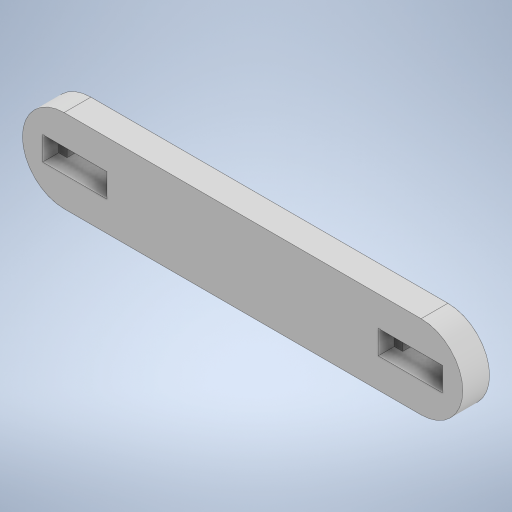
# Autodesk Inventor part: arm 2 right
Saved by Autodesk Inventor 2023 (Build 270158000, 158)
## iProperties
Created: 2024-06-28
Part Number: arm 2 right
Material: Generic
Document SubType Name: Modeling
Designer: Swoby
Density: 1 g/cm^3
Appearance: Default
Author: Swoby
Autodesk Inventor part; units mm, degrees
ref_plane "YZ Plane" through (0, 0, 0) normal (1, 0, 0) x (0, 1, 0)
ref_plane "XZ Plane" through (0, 0, 0) normal (0, 1, 0) x (-1, 0, 0)
ref_plane "XY Plane" through (0, 0, 0) normal (0, 0, 1) x (1, 0, 0)
sketch "Sketch1" plane through (0, 0, 0) normal (0, 0, 1) x (1, 0, 0)
  line L0 (-150, 0) -> (150, 0) construction
  line L1 (-150, -35) -> (150, -35)
  line L2 (150, 35) -> (-150, 35)
  arc A0 (-150, 35) -> (-150, -35) centre (-150, 0) ccw
  arc A1 (150, -35) -> (150, 35) centre (150, 0) ccw
  point P0 (0, 0)
  dimension "d0" = 150
  dimension "d1" = 70
  constraints: 8 end point, 4 point on circle, 4 tangent, 2 centre point, 1 horizontal, 1 midpoint, 1 parallel
  measures "d0" distance of point (0, 0) L0.end
  measures "d1" diameter of A1
extrude "Extrusion1" add sketch "Sketch1" along normal blind 22.5
sketch "Sketch2" plane through (0, 0, 22.5) normal (0, 0, 1) x (1, 0, 0)
  arc A0 (150, -35) -> (150, 35) centre (150, 0) ccw projected
  line L0 (114, 10) -> (168, 10)
  line L1 (168, 10) -> (168, -10)
  line L2 (168, -10) -> (114, -10)
  line L3 (114, -10) -> (114, 10)
  line L4 (121, 10) -> (161, 10)
  line L5 (161, 10) -> (161, -10)
  line L6 (161, -10) -> (121, -10)
  line L7 (121, -10) -> (121, 10)
  line L8 (114, 0) -> (121, 0)
  line L9 (0, 35) -> (0, -35)
  arc A1 (-150, 35) -> (-150, -35) centre (-150, 0) ccw
  line L10 (-114, 10) -> (-168, 10)
  line L11 (-168, 10) -> (-168, -10)
  line L12 (-168, -10) -> (-114, -10)
  line L13 (-114, -10) -> (-114, 10)
  line L14 (-121, 10) -> (-161, 10)
  line L15 (-161, 10) -> (-161, -10)
  line L16 (-161, -10) -> (-121, -10)
  line L17 (-121, -10) -> (-121, 10)
  line L18 (-114, 0) -> (-121, 0)
  point P0 (0, 0)
  point P1 (168, 0)
  point P2 (121, -10)
  point P3 (161, 10)
  point P4 (-168, 0)
  point P5 (-121, -10)
  point P6 (-161, 10)
  dimension "d4" = 54
  dimension "d5" = 40
  dimension "d6" = 7
  dimension "d7" = 20
  dimension "d8" = 36
  constraints: 38 end point, 14 symmetric about line, 6 point on line, 4 midpoint, 4 parallel, 2 horizontal, 2 perpendicular, 2 point on circle, 1 centre point, 1 vertical, 1 other
  measures "d4" distance of L0.start L0.end
  measures "d5" distance between parallel lines of L7 L5
  measures "d6" distance from line of point (168, 0) L5
  measures "d7" distance of L0.end L1.end
  measures "d8" distance of L8.start A0.centre
extrude "Extrusion2" cut sketch "Sketch2" against normal through all contours L0 L5 L2 L7 | L17 L12 L15 L10
extrude "Extrusion3" cut sketch "Sketch2" against normal blind 13.5 contours L0 L7 L8 L3 | L8 L7 L2 L3 | L0 L1 L2 L5 | L13 L18 L17 L10 | L13 L12 L17 L18 | L15 L12 L11 L10
body "Solid1"
